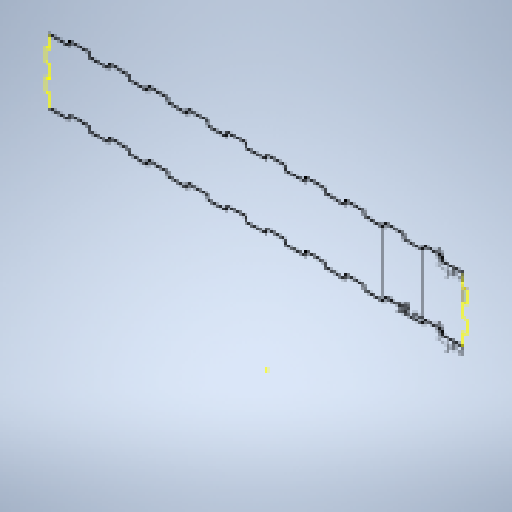
# Autodesk Inventor part: BackWall
Saved by Autodesk Inventor 2024 (Build 280153000, 153)
## iProperties
Created: 2023-09-10
Part Number: BackWall
Material: Generic
Document SubType Name: Modeling
Designer: Bruno
Density: 1 g/cm^3
Appearance: Default
Author: Bruno
Autodesk Inventor part; units mm, degrees
ref_plane "YZ Plane" through (0, 0, 0) normal (1, 0, 0) x (0, 1, 0)
ref_plane "XZ Plane" through (0, 0, 0) normal (0, 1, 0) x (-1, 0, 0)
ref_plane "XY Plane" through (0, 0, 0) normal (0, 0, 1) x (1, 0, 0)
ref_plane "Work Plane1" through (139.4467, 111.518, -98.9659) normal (0, 0, -1) x (-1, 0, 0)
sketch "Sketch1" plane through (139.4467, 111.518, -98.9659) normal (0, 0, -1) x (-1, 0, 0)
  line L0 (0, 9.125) -> (0, 18.25) projected
  line L1 (0, -9.125) -> (0, 0) projected
  line L2 (-3, -18.25) -> (-3, -9.125) projected
  line L3 (-3, 0) -> (-3, 9.125) projected
  line L4 (0, 0) -> (-3, 0) projected
  line L5 (0, -9.125) -> (-3, -9.125) projected
  line L6 (0, -18.25) -> (-3, -18.25) projected
  line L7 (0, -27.375) -> (0, -18.25) projected
  line L8 (0, 9.125) -> (-3, 9.125) projected
  line L9 (294, 9.125) -> (294, 18.25) projected
  line L10 (297, 0) -> (297, 9.125) projected
  line L11 (294, -9.125) -> (294, 0) projected
  line L12 (297, -18.25) -> (297, -9.125) projected
  line L13 (294, -27.375) -> (294, -18.25) projected
  line L14 (297, -18.25) -> (294, -18.25) projected
  line L15 (297, -9.125) -> (294, -9.125) projected
  line L16 (297, 0) -> (294, 0) projected
  line L17 (297, 9.125) -> (294, 9.125) projected
  line L18 (0, -27.375) -> (14, -27.375)
  line L19 (14, -27.375) -> (14, -24.375)
  line L20 (14, -24.375) -> (28, -24.375)
  line L21 (28, -24.375) -> (28, -27.375)
  line L22 (56, -24.375) -> (56, -27.375)
  line L23 (42, -24.375) -> (56, -24.375)
  line L24 (42, -27.375) -> (42, -24.375)
  line L25 (28, -27.375) -> (42, -27.375)
  line L26 (84, -24.375) -> (84, -27.375)
  line L27 (70, -24.375) -> (84, -24.375)
  line L28 (70, -27.375) -> (70, -24.375)
  line L29 (56, -27.375) -> (70, -27.375)
  line L30 (112, -24.375) -> (112, -27.375)
  line L31 (98, -24.375) -> (112, -24.375)
  line L32 (98, -27.375) -> (98, -24.375)
  line L33 (84, -27.375) -> (98, -27.375)
  line L34 (140, -24.375) -> (140, -27.375)
  line L35 (126, -24.375) -> (140, -24.375)
  line L36 (126, -27.375) -> (126, -24.375)
  line L37 (112, -27.375) -> (126, -27.375)
  line L38 (168, -24.375) -> (168, -27.375)
  line L39 (154, -24.375) -> (168, -24.375)
  line L40 (154, -27.375) -> (154, -24.375)
  line L41 (140, -27.375) -> (154, -27.375)
  line L42 (196, -24.375) -> (196, -27.375)
  line L43 (182, -24.375) -> (196, -24.375)
  line L44 (182, -27.375) -> (182, -24.375)
  line L45 (168, -27.375) -> (182, -27.375)
  line L46 (224, -24.375) -> (224, -27.375)
  line L47 (210, -24.375) -> (224, -24.375)
  line L48 (210, -27.375) -> (210, -24.375)
  line L49 (196, -27.375) -> (210, -27.375)
  line L50 (252, -24.375) -> (252, -27.375)
  line L51 (238, -24.375) -> (252, -24.375)
  line L52 (238, -27.375) -> (238, -24.375)
  line L53 (224, -27.375) -> (238, -27.375)
  line L54 (280, -24.375) -> (280, -27.375)
  line L55 (266, -24.375) -> (280, -24.375)
  line L56 (266, -27.375) -> (266, -24.375)
  line L57 (252, -27.375) -> (266, -27.375)
  line L58 (280, -27.375) -> (294, -27.375)
  line L59 (0, 18.25) -> (14, 18.25)
  line L60 (14, 18.25) -> (14, 21.25)
  line L61 (14, 21.25) -> (28, 21.25)
  line L62 (28, 21.25) -> (28, 18.25)
  line L63 (56, 21.25) -> (56, 18.25)
  line L64 (42, 21.25) -> (56, 21.25)
  line L65 (42, 18.25) -> (42, 21.25)
  line L66 (28, 18.25) -> (42, 18.25)
  line L67 (84, 21.25) -> (84, 18.25)
  line L68 (70, 21.25) -> (84, 21.25)
  line L69 (70, 18.25) -> (70, 21.25)
  line L70 (56, 18.25) -> (70, 18.25)
  line L71 (112, 21.25) -> (112, 18.25)
  line L72 (98, 21.25) -> (112, 21.25)
  line L73 (98, 18.25) -> (98, 21.25)
  line L74 (84, 18.25) -> (98, 18.25)
  line L75 (140, 21.25) -> (140, 18.25)
  line L76 (126, 21.25) -> (140, 21.25)
  line L77 (126, 18.25) -> (126, 21.25)
  line L78 (112, 18.25) -> (126, 18.25)
  line L79 (168, 21.25) -> (168, 18.25)
  line L80 (154, 21.25) -> (168, 21.25)
  line L81 (154, 18.25) -> (154, 21.25)
  line L82 (140, 18.25) -> (154, 18.25)
  line L83 (196, 21.25) -> (196, 18.25)
  line L84 (182, 21.25) -> (196, 21.25)
  line L85 (182, 18.25) -> (182, 21.25)
  line L86 (168, 18.25) -> (182, 18.25)
  line L87 (224, 21.25) -> (224, 18.25)
  line L88 (210, 21.25) -> (224, 21.25)
  line L89 (210, 18.25) -> (210, 21.25)
  line L90 (196, 18.25) -> (210, 18.25)
  line L91 (252, 21.25) -> (252, 18.25)
  line L92 (238, 21.25) -> (252, 21.25)
  line L93 (238, 18.25) -> (238, 21.25)
  line L94 (224, 18.25) -> (238, 18.25)
  line L95 (280, 21.25) -> (280, 18.25)
  line L96 (266, 21.25) -> (280, 21.25)
  line L97 (266, 18.25) -> (266, 21.25)
  line L98 (252, 18.25) -> (266, 18.25)
  line L99 (280, 18.25) -> (294, 18.25)
  point P0 (139.4467, -111.518)
  point P1 (28, -27.375)
  point P2 (56, -27.375)
  point P3 (168, -27.375)
  point P4 (224, -27.375)
  point P5 (252, 18.25)
  point P6 (224, 18.25)
  point P7 (196, 18.25)
  point P8 (168, 18.25)
  point P9 (140, 18.25)
  point P10 (112, 18.25)
  point P11 (84, 18.25)
  point P12 (56, 18.25)
  point P13 (28, 18.25)
  point P14 (0, 18.25)
  dimension "d0" = 3
  dimension "d1" = 14
  dimension "d4" = 28
  dimension "d13" = 3
  dimension "d14" = 14
  dimension "d15" = 28
  constraints: 164 end point, 20 point on line, 6 horizontal, 6 perpendicular, 2 collinear, 2 parallel, 1 coincident, 160 other
  measures "d0" distance of L18.end L19.end
  measures "d1" distance of L7.start L18.end
  measures "d4" distance of L20.end L22.start
  measures "d13" distance of L60.start L61.start
  measures "d14" distance of L59.start L60.start
  measures "d15" distance of L62.start L64.end
extrude "Extrusion1" add sketch "Sketch1" along normal blind 3
body "Solid1"
